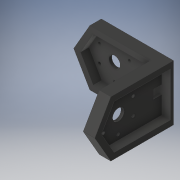
# Autodesk Inventor part: TARM03
Saved by Autodesk Inventor 2017 (Build 210142000, 142)
## iProperties
Created: 2018-10-19
Part Number: TARM03
Material: ABS Plastic
Document SubType Name: Modeling
Designer: Dell
Density: 1.06 g/cm^3
Appearance: Smooth - Black
Author: Dell
Autodesk Inventor part; units mm, degrees
ref_plane "YZ Plane" through (0, 0, 0) normal (1, 0, 0) x (0, 1, 0)
ref_plane "XZ Plane" through (0, 0, 0) normal (0, 1, 0) x (-1, 0, 0)
ref_plane "XY Plane" through (0, 0, 0) normal (0, 0, 1) x (1, 0, 0)
sketch "Sketch1" plane through (0, 0, 0) normal (0, 0, 1) x (1, 0, 0)
  line L0 (-56, 0) -> (-28, 48.4974)
  line L1 (-28, 48.4974) -> (28, 48.4974)
  line L2 (28, 48.4974) -> (56, 0)
  line L3 (56, 0) -> (28, -48.4974)
  line L4 (28, -48.4974) -> (-28, -48.4974)
  line L5 (-28, -48.4974) -> (-56, 0)
  circle A0 centre (0, 30) radius 2.5
  circle A1 centre (-25.9808, 15) radius 2.5
  circle A2 centre (-25.9808, -15) radius 2.5
  circle A3 centre (0, -30) radius 2.5
  circle A4 centre (25.9808, -15) radius 2.5
  circle A5 centre (25.9808, 15) radius 2.5
  point P0 (0, 0)
  point P1 (0, 0)
  dimension "d0" = 112
  dimension "d1" = 5
  dimension "d2" = 30
  dimension "d5" = 360
  constraints: 12 end point, 6 centre point, 1 coincident, 1 horizontal alignment, 1 vertical alignment, 26 other
  measures "d0" distance of L2.end L0.start
  measures "d1" diameter of A0
  measures "d2" distance of point (0, 0) A0.centre
extrude "Extrusion1" add sketch "Sketch1" along normal blind 5
sketch "Sketch2" plane through (0, 0, 5) normal (0, 0, 1) x (1, 0, 0)
  line L0 (28, 48.4974) -> (-28, 48.4974) projected
  line L1 (28, 48.4974) -> (82.5, 48.4974)
  line L2 (82.5, 48.4974) -> (82.5, -48.4974)
  line L3 (82.5, -48.4974) -> (28, -48.4974)
  circle A0 centre (25.9808, 15) radius 2.5 projected
  circle A1 centre (25.9808, -15) radius 2.5 projected
  line L4 (56, 0) -> (28, 48.4974) projected
  line L5 (28, -48.4974) -> (56, 0) projected
  line L6 (-28, -48.4974) -> (28, -48.4974) projected
  line L7 (28, -48.4974) -> (56, 0)
  line L8 (28, 48.4974) -> (56, 0)
  line L9 (28, -48.4974) -> (82.5, -48.4974)
  line L10 (28, 48.4974) -> (82.5, 48.4974)
  point P0 (0, 0)
  dimension "d42" = 82.5
  constraints: 14 end point, 3 equal length, 1 horizontal, 1 horizontal alignment, 1 perpendicular
  measures "d42" distance from line of point (0, 0) L2
extrude "Extrusion2" add sketch "Sketch2" against normal blind 5 contours L1 L2 L3 L5 L4
sketch "Sketch3" plane through (82.5, -48.4974, 5) normal (1, 0, 0) x (0, 0, -1)
  line L0 (0, 0) -> (0, 96.9948) projected
  line L1 (-48, 96.9948) -> (-20, 48.4974)
  line L2 (-20, 48.4974) -> (-48, 0)
  line L3 (-48, 0) -> (-104, 0)
  line L4 (-104, 0) -> (-132, 48.4974)
  line L5 (-132, 48.4974) -> (-104, 96.9948)
  line L6 (-104, 96.9948) -> (-48, 96.9948)
  line L7 (0, 0) -> (-48, 0)
  line L8 (-48, 0) -> (-48, 96.9948) construction
  line L9 (-48, 96.9948) -> (0, 96.9948)
  line L10 (0, 96.9948) -> (0, 0)
  circle A0 centre (-76, 78.4974) radius 2.5
  circle A1 centre (-101.9808, 63.4974) radius 2.5
  circle A2 centre (-101.9808, 33.4974) radius 2.5
  circle A3 centre (-76, 18.4974) radius 2.5
  circle A4 centre (-50.0192, 33.4974) radius 2.5
  circle A5 centre (-50.0192, 63.4974) radius 2.5
  line L11 (-48, 0) -> (-20, 48.4974)
  line L12 (-20, 48.4974) -> (-48, 96.9948)
  line L13 (-48, 96.9948) -> (0, 96.9948)
  line L14 (0, 48.4974) -> (0, 0) projected
  line L15 (-48, 0) -> (0, 0)
  circle A6 centre (-76, 48.4974) radius 10
  point P0 (5, 48.4974)
  dimension "d17" = 112
  dimension "d18" = 20
  dimension "d19" = 5
  dimension "d20" = 30
  dimension "d23" = 360
  dimension "d27" = 20
  constraints: 28 end point, 7 centre point, 4 equal length, 3 horizontal, 1 coincident, 1 perpendicular, 1 vertical alignment, 26 other
  measures "d17" distance of L1.end L4.end
  measures "d18" distance from line of L0 L1.end
  measures "d19" diameter of A0
  measures "d20" distance of A0.centre point (-76, 48.497)
  measures "d27" diameter of A6
extrude "Extrusion3" add sketch "Sketch3" against normal blind 5
sketch "Sketch4" plane through (0, 0, 5) normal (0, 0, 1) x (1, 0, 0)
  circle A0 centre (0, 0) radius 10
  dimension "d28" = 20
  constraints: 1 centre point, 1 coincident
  measures "d28" diameter of A0
extrude "Extrusion4" cut sketch "Sketch4" against normal through all
sketch "Sketch5" plane through (0, 0, 5) normal (0, 0, 1) x (1, 0, 0)
  circle A0 centre (0, 0) radius 10 projected
  line L0 (77.5, -48.4974) -> (77.5, 48.4974) construction
  line L1 (77.5, 48.4974) -> (-28, 48.4974) projected
  line L2 (-28, 48.4974) -> (-56, 0) projected
  line L3 (-56, 0) -> (-28, -48.4974) projected
  line L4 (-28, -48.4974) -> (77.5, -48.4974) projected
  circle A1 centre (25.9808, 15) radius 2.5 projected
  circle A2 centre (25.9808, -15) radius 2.5 projected
  circle A3 centre (0, -30) radius 2.5 projected
  circle A4 centre (-25.9808, -15) radius 2.5 projected
  circle A5 centre (-25.9808, 15) radius 2.5 projected
  circle A6 centre (0, 30) radius 2.5 projected
  line L5 (-22.2265, 38.4974) -> (67.5, 38.4974)
  line L6 (67.5, 38.4974) -> (67.5, -38.4974) construction
  line L7 (67.5, -38.4974) -> (-22.2265, -38.4974)
  line L8 (-22.2265, -38.4974) -> (-44.453, 0)
  line L9 (-44.453, 0) -> (-22.2265, 38.4974)
  line L10 (67.5, 38.4974) -> (77.5, 38.4974)
  line L11 (77.5, -48.4974) -> (77.5, 48.4974) projected
  line L12 (77.5, 48.4974) -> (77.5, 38.4974)
  line L13 (67.5, -38.4974) -> (77.5, -38.4974)
  line L14 (77.5, -38.4974) -> (77.5, -48.4974)
  dimension "d31" = 10
  constraints: 18 end point, 2 collinear, 2 perpendicular, 2 point on line, 4 other
  measures "d31" distance between parallel lines of L1 L5
extrude "Extrusion5" add sketch "Sketch5" along normal blind 15 contours L11 L10 L5 L9 L8 L7 L13 L4 L3 L2 L1
sketch "Sketch7" plane through (77.5, -48.4974, 5) normal (-1, 0, 0) x (0, 0, 1)
  circle A0 centre (76, 78.4974) radius 2.5 projected
  circle A1 centre (101.9808, 63.4974) radius 2.5 projected
  circle A2 centre (101.9808, 33.4974) radius 2.5 projected
  circle A3 centre (76, 18.4974) radius 2.5 projected
  circle A4 centre (50.0192, 33.4974) radius 2.5 projected
  circle A5 centre (50.0192, 63.4974) radius 2.5 projected
  circle A6 centre (76, 48.4974) radius 10 projected
  line L0 (15, 96.9948) -> (15, 86.9948) projected
  line L1 (15, 86.9948) -> (0, 86.9948) projected
  line L2 (0, 10) -> (0, 86.9948) projected
  line L3 (0, 10) -> (15, 10) projected
  line L4 (15, 10) -> (15, 0) projected
  line L5 (15, 0) -> (104, 0) projected
  line L6 (104, 0) -> (132, 48.4974) projected
  line L7 (132, 48.4974) -> (104, 96.9948) projected
  line L8 (104, 96.9948) -> (15, 96.9948) projected
  line L9 (0, 55.9974) -> (15, 55.9974)
  line L10 (15, 55.9974) -> (15, 40.9974)
  line L11 (15, 40.9974) -> (0, 40.9974)
  line L12 (0, 40.9974) -> (0, 55.9974)
  point P0 (-5, 48.4974)
  point P1 (0, 48.4974)
  dimension "d34" = 15
  constraints: 8 end point, 2 midpoint, 2 parallel, 1 horizontal, 1 perpendicular, 1 point on line, 1 vertical alignment
  measures "d34" distance of L9.end L10.end
extrude "Extrusion6" cut sketch "Sketch7" against normal through all contours L9 L10 L11 L2
sketch "Sketch8" plane through (82.5, -48.4974, 0) normal (1, 0, 0) x (0, 0, -1)
  line L0 (-5, 40.9974) -> (-20, 40.9974) projected
  line L1 (-20, 40.9974) -> (-20, 55.9974) projected
  line L2 (-20, 55.9974) -> (-5, 55.9974) projected
  line L3 (-5, 55.9974) -> (-5, 40.9974) projected
  circle A0 centre (-81, 78.4974) radius 2.5 projected
  circle A1 centre (-106.9808, 63.4974) radius 2.5 projected
  circle A2 centre (-106.9808, 33.4974) radius 2.5 projected
  circle A3 centre (-81, 18.4974) radius 2.5 projected
  circle A4 centre (-55.0192, 33.4974) radius 2.5 projected
  circle A5 centre (-55.0192, 63.4974) radius 2.5 projected
  circle A6 centre (-81, 48.4974) radius 10 projected
  line L4 (-109, 0) -> (0, 0) projected
  line L5 (0, 96.9948) -> (0, 0) projected
  line L6 (0, 96.9948) -> (-109, 96.9948) projected
  line L7 (-109, 96.9948) -> (-137, 48.4974) projected
  line L8 (-137, 48.4974) -> (-109, 0) projected
  line L9 (-103.2265, 86.9948) -> (-10, 86.9948)
  line L10 (-10, 86.9948) -> (-10, 10) construction
  line L11 (-10, 10) -> (-103.2265, 10)
  line L12 (-103.2265, 10) -> (-125.453, 48.4974)
  line L13 (-125.453, 48.4974) -> (-103.2265, 86.9948)
  line L14 (-10, 86.9948) -> (0, 86.9948)
  line L15 (-10, 10) -> (0, 10)
  line L16 (0, 96.9948) -> (0, 0) projected
  point P0 (0, 48.4974)
  dimension "d37" = 10
  constraints: 14 end point, 2 point on line, 1 horizontal, 1 perpendicular, 4 other
  measures "d37" distance between parallel lines of L6 L9
extrude "Extrusion7" add sketch "Sketch8" along normal blind 15 contours L8 L7 L6 L5 L14 L9 L13 L12 L11 L15 L4
sketch "Sketch9" plane through (82.5, -38.4974, 0) normal (1, 0, 0) x (0, 0, -1)
  line L0 (0, 76.9948) -> (0, 86.9948) projected
  line L1 (0, 76.9948) -> (-5, 76.9948)
  line L2 (-5, 76.9948) -> (-5, -0.838)
  line L3 (-5, -0.838) -> (0, -0.838)
  line L4 (0, -0.838) -> (0, 76.9948)
  line L5 (-5, 45.9974) -> (-5, 30.9974) projected
  point P0 (0, 38.4974)
  constraints: 8 end point, 2 parallel, 1 horizontal, 1 perpendicular, 1 point on line
extrude "Extrusion8" add sketch "Sketch9" along normal blind 15
equation "\"d29\" = d28"
body "Solid1"
